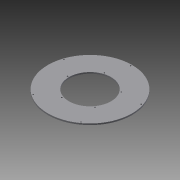
# Autodesk Inventor part: bakplate
Saved by Autodesk Inventor 2015 (Build 190159000, 159)
## iProperties
Created: 2015-02-04
Part Number: bakplate
Material: Generic
Document SubType Name: Modeling
Designer: janov_000
Density: 1 g/cm^3
Appearance: Aluminum - Flat
od: 320,000 mm
id: 150,000 mm
Author: janov_000
Autodesk Inventor part; units mm, degrees
ref_plane "YZ Plane" through (0, 0, 0) normal (1, 0, 0) x (0, 1, 0)
ref_plane "XZ Plane" through (0, 0, 0) normal (0, 1, 0) x (-1, 0, 0)
ref_plane "XY Plane" through (0, 0, 0) normal (0, 0, 1) x (1, 0, 0)
sketch "Sketch1" plane through (0, 0, 0) normal (0, 0, 1) x (1, 0, 0)
  circle A0 centre (0, 0) radius 75
  circle A1 centre (0, 0) radius 160
  dimension "inner_diameter" = 150
  dimension "outer_diameter" = 320
  constraints: 2 centre point, 2 coincident
  measures "inner_diameter" diameter of A0
  measures "outer_diameter" diameter of A1
extrude "Extrusion1" add sketch "Sketch1" along normal blind 5
sketch "Sketch2" plane through (0, 0, 5) normal (0, 0, 1) x (1, 0, 0)
  circle A0 centre (0, 0) radius 155 construction
  line L0 (0.1758, 0.0573) -> (40.2666, 149.6783) construction
  line L1 (0.1758, 0.0573) -> (-129.7335, 84.4214) construction
  line L2 (0.1758, 0.0573) -> (-120.2034, -97.4238) construction
  line L3 (0.1758, 0.0573) -> (55.6866, -144.5534) construction
  line L4 (0.1758, 0.0573) -> (154.8625, 8.1641) construction
  line L5 (0.1758, 0.0573) -> (0.1758, 154.9999) construction
  dimension "d4" = 310
  dimension "d30" = 360
  dimension "d36" = 15
  constraints: 12 end point, 8 coincident, 2 point on circle, 1 centre point, 1 vertical, 20 other
  measures "d4" diameter of A0
  measures "d36" angle of L5 L0
hole "Hole1" at (40.2666, 149.6783, 5) at (-129.7335, 84.4214, 5) at (-120.2034, -97.4238, 5) at (55.6866, -144.5534, 5) at (154.8625, 8.1641, 5) direction (0, 0, -1) diameter 4.134 depth 8 tip angle 118 thread size "M5x0.8" class "6H" standard "ANSI Metric M Profile"
sketch "Sketch3" plane through (0, 0, 5) normal (0, 0, 1) x (1, 0, 0)
  circle A0 centre (0, 0) radius 80 construction
  line L0 (0, 0) -> (0, 80) construction
  point P0 (-76.0845, 24.7214)
  point P1 (-76.0845, 24.7214)
  point P2 (-47.0228, -64.7214)
  point P3 (-47.0228, -64.7214)
  point P4 (47.0228, -64.7214)
  point P5 (47.0228, -64.7214)
  point P6 (76.0845, 24.7214)
  point P7 (76.0845, 24.7214)
  dimension "inner_holes_diameter" = 160
  dimension "d34" = 360
  constraints: 12 coincident, 2 end point, 1 vertical, 1 vertical alignment, 21 other
hole "Hole2" at (0, 80, 5) at (76.0845, 24.7214, 5) at (47.0228, -64.7214, 5) at (-47.0228, -64.7214, 5) at (-76.0845, 24.7214, 5) direction (0, 0, -1) diameter 4.134 depth 8 tip angle 118 thread size "M5x0.8" class "6H" standard "ANSI Metric M Profile"
equation "\"inner_diameter\" = id"
equation "\"outer_diameter\" = od"
equation "\"id\" = 150"
equation "\"od\" = 320"
body "Solid1"
